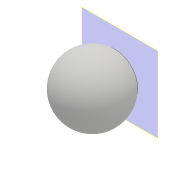
# Autodesk Inventor part: end_pad
Saved by Autodesk Inventor 2017 (Build 210142000, 142)
## iProperties
Created: 2018-05-30
Part Number: end_pad
Material: Generic
Document SubType Name: Modeling
Designer: Nic
Density: 1 g/cm^3
Appearance: Default
Author: Nic
Autodesk Inventor part; units mm, degrees
ref_plane "YZ Plane" through (0, 0, 0) normal (1, 0, 0) x (0, 1, 0)
ref_plane "XY Plane" through (0, 0, 0) normal (0, 0, 1) x (1, 0, 0)
sketch "Sketch1" plane through (0, 0, 0) normal (0, 0, 1) x (1, 0, 0)
  arc A0 (0, -14) -> (0, 14) centre (0, 0) ccw
  line L0 (0, 14) -> (0, -14)
  dimension "d0" = 28
  constraints: 2 end point, 2 point on circle, 1 centre point, 1 coincident, 1 midpoint, 1 vertical
  measures "d0" diameter of A0
revolve "Revolution1" add sketch "Sketch1" angle 360 about axis through (0, 14, 0) along (0, -1, 0)
sketch "Sketch2" plane through (0, 0, 0) normal (0, 0, 1) x (1, 0, 0)
  arc A0 (-9, 17) -> (9, 17) centre (0, 17) ccw
  line L0 (-9, 17) -> (9, 17)
  point P0 (0, 0)
  dimension "d2" = 17
  dimension "d13" = 9
  dimension "d19" = 18
  constraints: 2 end point, 2 point on circle, 1 centre point, 1 horizontal, 1 midpoint, 1 vertical alignment
  measures "d2" distance of point (0, 0) A0.centre
  measures "d13" radius of A0
  measures "d19" distance of L0.start L0.end
revolve "Revolution2" cut sketch "Sketch2" angle 360 about axis through (-9, 17, 0) along (1, 0, 0)
ref_plane "Work Plane2" through (0, 12, 0) normal (0, 1, 0) x (-1, 0, 0)
sketch "Sketch4" plane through (0, 12, 0) normal (0, 1, 0) x (-1, 0, 0)
  circle A0 centre (0, 0) radius 10
  dimension "d21" = 20
  constraints: 1 centre point, 1 coincident
  measures "d21" diameter of A0
extrude "Extrusion2" cut sketch "Sketch4" against normal blind 2
body "Solid1"
